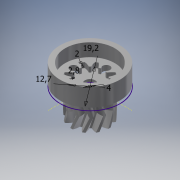
# Autodesk Inventor part: Stirnzahnrad1
Saved by Autodesk Inventor 2019.1 (Build 231200000, 200)
## iProperties
Created: 2018-07-09
Part Number: Stirnzahnrad1
Material: Steel
Document SubType Name: Modeling
Designer: JochenAlt
Categories: <?xml version="1.0" encoding="UTF-16"?> <MemberInstance><Categories><FamilyTemplate><FamilyTemplateParameter ValueType="xs:double" Id="1" ObjectReferenceKey="da_z" ObjectType="kUserParameterObject"/><FamilyTemplateParameter ValueType="xs:double" Id="2" ObjectReferenceKey="da_b" ObjectType="kUserParameterObject"/><FamilyTemplateParameter ValueType="xs:double" Id="3" ObjectReferenceKey="da_beta" ObjectType="kUserParameterObject"/><FamilyTemplateParameter ValueType="xs:double" Id="4" ObjectReferenceKey="da_da" ObjectType="kUserParameterObject"/><FamilyTemplateParameter ValueType="xs:double" Id="5" ObjectReferenceKey="da_aw" ObjectType="kUserParameterObject"/><FamilyTemplateParameter ValueType="xs:string" Id="6" ObjectReferenceKey="EAIAABAAAACIAQAAAAAAAIAAAAAAAAAA" ObjectType="83910656" SubObjectId="SurfaceGeometry"/></FamilyTemplate><ParamToTemplateMap><ParamToTemplate CategoryParameter="//CategoryParameter[@InternalName='046C89C9-8512-4d59-83FE-43B91F4F132A']" TemplateParameter="1"/><ParamToTemplate CategoryParameter="//CategoryParameter[@InternalName='2552DF32-E462-4b46-AEBF-C6C7768E72AC']" TemplateParameter="2"/><ParamToTemplate CategoryParameter="//CategoryParameter[@InternalName='C9EE641D-15FC-4fae-A226-E94C4372FDD7']" TemplateParameter="3"/><ParamToTemplate><ParamToTemplate CategoryParameter="//CategoryParameter[@InternalName='00B6519A-459B-49c7-AD84-2E56D39A5744']" ConstantValue="0.000000"/></ParamToTemplate><ParamToTemplate><ParamToTemplate CategoryParameter="//CategoryParameter[@InternalName='04B31F0E-C7A6-4894-AA32-9629BEFACF47']" ConstantValue="1.000000"/></ParamToTemplate><ParamToTemplate><ParamToTemplate CategoryParameter="//CategoryParameter[@InternalName='43CBEC2E-7847-49e7-A936-2F7889FCB2D9']" ConstantValue="0.250000"/></ParamToTemplate><ParamToTemplate><ParamToTemplate CategoryParameter="//CategoryParameter[@InternalName='B1EFC894-105D-4ebd-86BF-FA20ED196853']" ConstantValue="0.350000"/></ParamToTemplate><ParamToTemplate><ParamToTemplate CategoryParameter="//CategoryParameter[@InternalName='51175063-3D10-4879-93E8-6246FE8B403D']" ConstantValue="2060000000.000000"/></ParamToTemplate><ParamToTemplate><ParamToTemplate CategoryParameter="//CategoryParameter[@InternalName='A3A52E27-4454-46a9-B0BD-C932399B70AF']" ConstantValue="0.300000"/></ParamToTemplate><ParamToTemplate><ParamToTemplate CategoryParameter="//CategoryParameter[@InternalName='91B76062-C214-41d9-B1B9-14D2AB99603D']" ConstantValue="0.100000"/></ParamToTemplate><ParamToTemplate><ParamToTemplate CategoryParameter="//CategoryParameter[@InternalName='374E806E-8B8A-4dda-A9AA-1039D6500AD2']" ConstantValue="10.000000"/></ParamToTemplate><ParamToTemplate><ParamToTemplate CategoryParameter="//CategoryParameter[@InternalName='2D373A89-B862-43d6-8D0B-0CBF12AB9F6C']" ConstantValue="0.349066"/></ParamToTemplate><ParamToTemplate CategoryParameter="//CategoryParameter[@InternalName='37777632-D6A2-4fac-9D53-DB8ACD95C989']" TemplateParameter="4"/><ParamToTemplate CategoryParameter="//CategoryParameter[@InternalName='FD1017F1-B727-4f7e-9707-0F86F1FF9423']" TemplateParameter="5"/><ParamToTemplate><ParamToTemplate CategoryParameter="//CategoryParameter[@InternalName='9E1B4470-B2D3-4ff1-B813-535BB4CDF51A']" ConstantValue="3520000.000000"/></ParamToTemplate><ParamToTemplate><ParamToTemplate CategoryParameter="//CategoryParameter[@InternalName='F8452263-BFF6-458c-9FB1-07C4B99E95CD']" ConstantValue="11400000.000000"/></ParamToTemplate><ParamToTemplate><ParamToTemplate CategoryParameter="//CategoryParameter[@InternalName='3E3BB259-FD49-497f-8171-6EBC954A3479']" ConstantValue="2.000000"/></ParamToTemplate><ParamToTemplate CategoryParameter="//CategoryParameter[@InternalName='27C3BAF2-7550-4e4b-AE2C-0DB134B7D9B7']" TemplateParameter="6"/></ParamToTemplateMap><Category DisplayName="Gear" InternalName="DC85795E-93AB-48d5-8EEE-5A27447B64BD" Mnemonic="Gear"><CategoryParameter DisplayName="z" InternalName="046C89C9-8512-4d59-83FE-43B91F4F132A" Mnemonic="z"/><CategoryParameter DisplayName="b" InternalName="2552DF32-E462-4b46-AEBF-C6C7768E72AC" Mnemonic="b"/><CategoryParameter DisplayName="||b|" InternalName="C9EE641D-15FC-4fae-A226-E94C4372FDD7" Mnemonic="beta"/><CategoryParameter DisplayName="x" InternalName="00B6519A-459B-49c7-AD84-2E56D39A5744" Mnemonic="x"/><CategoryParameter DisplayName="a*" InternalName="04B31F0E-C7A6-4894-AA32-9629BEFACF47" Mnemonic="a"/><CategoryParameter DisplayName="c*" InternalName="43CBEC2E-7847-49e7-A936-2F7889FCB2D9" Mnemonic="c"/><CategoryParameter DisplayName="r|.f|*" InternalName="B1EFC894-105D-4ebd-86BF-FA20ED196853" Mnemonic="rf"/><CategoryParameter DisplayName="E" InternalName="51175063-3D10-4879-93E8-6246FE8B403D" Mnemonic="E"/><CategoryParameter DisplayName="||m|" InternalName="A3A52E27-4454-46a9-B0BD-C932399B70AF" Mnemonic="mi"/><Category DisplayName="SpurGear" InternalName="26C5A22E-A91E-4dfd-A3B3-23CCAFAE1764" Mnemonic="SpurGear"><CategoryParameter DisplayName="m" InternalName="91B76062-C214-41d9-B1B9-14D2AB99603D" Mnemonic="m"/><CategoryParameter DisplayName="P" InternalName="374E806E-8B8A-4dda-A9AA-1039D6500AD2" Mnemonic="PP"/><CategoryParameter DisplayName="||a|" InternalName="2D373A89-B862-43d6-8D0B-0CBF12AB9F6C" Mnemonic="alpha"/><CategoryParameter DisplayName="d|.a|" InternalName="37777632-D6A2-4fac-9D53-DB8ACD95C989" Mnemonic="da"/><CategoryParameter DisplayName="a|.w|" InternalName="FD1017F1-B727-4f7e-9707-0F86F1FF9423" Mnemonic="aw"/><CategoryParameter DisplayName="||s||.Flim|" InternalName="9E1B4470-B2D3-4ff1-B813-535BB4CDF51A" Mnemonic="sFlim"/><CategoryParameter DisplayName="||s||.Hlim|" InternalName="F8452263-BFF6-458c-9FB1-07C4B99E95CD" Mnemonic="sHlim"/><CategoryParameter DisplayName="Typ" InternalName="3E3BB259-FD49-497f-8171-6EBC954A3479" Mnemonic="type"/><CategoryParameter DisplayName="PitchDiameter" InternalName="27C3BAF2-7550-4e4b-AE2C-0DB134B7D9B7" Mnemonic="IDS_PITCHDIAM"/></Category></Category></Categories></MemberInstance>
Density: 1 g/cm^3
Appearance: Steel
CustomPartVersion: 1
Author: JochenAlt
Autodesk Inventor part; units mm, degrees
sketch "Sketch1" plane through (0, 0, 0) normal (0, 0, 1) x (1, 0, 0)
  circle A0 centre (0, 0) radius 7.3851
  dimension "d0" = 14.7701
  constraints: 1 centre point
  measures "d0" diameter of A0
extrude "Extrusion1" add sketch "Sketch1" along normal blind 5.5
ref_plane "Work Plane2" through (0, 0, 2.75) normal (0, 0, 1) x (1, 0, 0)
sketch "Sketch2" plane through (0, 0, 0) normal (0, 0, -1) x (-1, 0, 0)
  circle A0 centre (0, 0) radius 7.3851 projected
  circle A1 centre (0, 0) radius 6.375
  dimension "d3" = 12.75
  constraints: 1 centre point, 1 coincident
  measures "d3" diameter of A1
surface extrude "Flankendurchmesser" sketch "Sketch2" against normal through all shown no curves A1
ref_plane "Work Plane8" through (0, 0, 0) normal (0.9659258, 0.258819, 0) x (0, 0, 1)
ref_plane "Work Plane9" through (0, 0, 0) normal (1, 0, 0) x (0, 1, 0)
spur gear teeth "Stirnzahnrad" teeth 12 pitch diameter 12.7701 tip diameter 14.7701 root diameter 10.2701 face width 5.5 helix angle 20 hand right start plane through (0, 0, 0) normal (0, 0, -1) x (-1, 0, 0)
mirror "Spiegeln2" about plane through (0, 0, 5.5) normal (0, 0, 1)
sketch "Skizze3" plane through (0, 0, 11) normal (0, 0, 1) x (1, 0, 0)
  circle A0 centre (0, 0) radius 2
  circle A1 centre (0, 0) radius 9.6
  circle A2 centre (0, 0) radius 11.6
  circle A3 centre (0, 0) radius 6.35 construction
  circle A4 centre (-6.35, 0) radius 1.4
  circle A5 centre (6.35, 0) radius 1.4
  circle A6 centre (0, 6.35) radius 1.4
  circle A7 centre (0, -6.35) radius 1.4
  line L0 (0, 16.24) -> (0, -16.24) construction
  line L1 (-16.24, 0) -> (16.24, 0) construction
  spline S0 degree 5 poles (-3.3858, 3.8607) (-3.6167, 4.2827) (-3.8063, 4.7273) (-3.9516, 5.1892) (-4.0507, 5.6623) (-4.1029, 6.1405) knots 0 0 0 0 0 0 1 1 1 1 1 1 projected
  spline S1 degree 5 poles (-3.8607, 3.3858) (-3.7721, 3.4869) (-3.6802, 3.585) (-3.585, 3.6802) (-3.4869, 3.7721) (-3.3858, 3.8607) knots 0 0 0 0 0 0 1 1 1 1 1 1 projected
  spline S2 degree 5 poles (-6.1405, 4.1029) (-5.6623, 4.0507) (-5.1892, 3.9516) (-4.7273, 3.8063) (-4.2827, 3.6167) (-3.8607, 3.3858) knots 0 0 0 0 0 0 1 1 1 1 1 1 projected
  arc A8 (-6.1405, 4.1029) -> (-6.6235, 3.2663) centre (0, 0) ccw projected
  spline S3 degree 5 poles (-4.8625, 1.6506) (-5.2735, 1.9006) (-5.66, 2.1909) (-6.0168, 2.5182) (-6.3391, 2.8783) (-6.6235, 3.2663) knots 0 0 0 0 0 0 1 1 1 1 1 1 projected
  spline S4 degree 5 poles (-5.0364, 1.0018) (-5.0102, 1.1337) (-4.9796, 1.2646) (-4.9448, 1.3946) (-4.9058, 1.5233) (-4.8625, 1.6506) knots 0 0 0 0 0 0 1 1 1 1 1 1 projected
  spline S5 degree 5 poles (-7.3693, 0.483) (-6.929, 0.6769) (-6.4698, 0.8276) (-5.9972, 0.9327) (-5.5173, 0.9908) (-5.0364, 1.0018) knots 0 0 0 0 0 0 1 1 1 1 1 1 projected
  arc A9 (-7.3693, 0.483) -> (-7.3693, -0.483) centre (0, 0) ccw projected
  spline S6 degree 5 poles (-5.0364, -1.0018) (-5.5173, -0.9908) (-5.9972, -0.9327) (-6.4698, -0.8276) (-6.929, -0.6769) (-7.3693, -0.483) knots 0 0 0 0 0 0 1 1 1 1 1 1 projected
  spline S7 degree 5 poles (-4.8625, -1.6506) (-4.9058, -1.5233) (-4.9448, -1.3946) (-4.9796, -1.2646) (-5.0102, -1.1337) (-5.0364, -1.0018) knots 0 0 0 0 0 0 1 1 1 1 1 1 projected
  spline S8 degree 5 poles (-6.6235, -3.2663) (-6.3391, -2.8783) (-6.0168, -2.5182) (-5.66, -2.1909) (-5.2735, -1.9006) (-4.8625, -1.6506) knots 0 0 0 0 0 0 1 1 1 1 1 1 projected
  arc A10 (-6.6235, -3.2663) -> (-6.1405, -4.1029) centre (0, 0) ccw projected
  spline S9 degree 5 poles (-3.8607, -3.3858) (-4.2827, -3.6167) (-4.7273, -3.8063) (-5.1892, -3.9516) (-5.6623, -4.0507) (-6.1405, -4.1029) knots 0 0 0 0 0 0 1 1 1 1 1 1 projected
  spline S10 degree 5 poles (-3.3858, -3.8607) (-3.4869, -3.7721) (-3.585, -3.6802) (-3.6802, -3.585) (-3.7721, -3.4869) (-3.8607, -3.3858) knots 0 0 0 0 0 0 1 1 1 1 1 1 projected
  spline S11 degree 5 poles (-4.1029, -6.1405) (-4.0507, -5.6623) (-3.9516, -5.1892) (-3.8063, -4.7273) (-3.6167, -4.2827) (-3.3858, -3.8607) knots 0 0 0 0 0 0 1 1 1 1 1 1 projected
  arc A11 (-4.1029, -6.1405) -> (-3.2663, -6.6235) centre (0, 0) ccw projected
  spline S12 degree 5 poles (-1.6506, -4.8625) (-1.9006, -5.2735) (-2.1909, -5.66) (-2.5182, -6.0168) (-2.8783, -6.3391) (-3.2663, -6.6235) knots 0 0 0 0 0 0 1 1 1 1 1 1 projected
  spline S13 degree 5 poles (-1.0018, -5.0364) (-1.1337, -5.0102) (-1.2646, -4.9796) (-1.3946, -4.9448) (-1.5233, -4.9058) (-1.6506, -4.8625) knots 0 0 0 0 0 0 1 1 1 1 1 1 projected
  spline S14 degree 5 poles (-0.483, -7.3693) (-0.6769, -6.929) (-0.8276, -6.4698) (-0.9327, -5.9972) (-0.9908, -5.5173) (-1.0018, -5.0364) knots 0 0 0 0 0 0 1 1 1 1 1 1 projected
  arc A12 (-0.483, -7.3693) -> (0.483, -7.3693) centre (0, 0) ccw projected
  spline S15 degree 5 poles (1.0018, -5.0364) (0.9908, -5.5173) (0.9327, -5.9972) (0.8276, -6.4698) (0.6769, -6.929) (0.483, -7.3693) knots 0 0 0 0 0 0 1 1 1 1 1 1 projected
  spline S16 degree 5 poles (1.6506, -4.8625) (1.5233, -4.9058) (1.3946, -4.9448) (1.2646, -4.9796) (1.1337, -5.0102) (1.0018, -5.0364) knots 0 0 0 0 0 0 1 1 1 1 1 1 projected
  spline S17 degree 5 poles (3.2663, -6.6235) (2.8783, -6.3391) (2.5182, -6.0168) (2.1909, -5.66) (1.9006, -5.2735) (1.6506, -4.8625) knots 0 0 0 0 0 0 1 1 1 1 1 1 projected
  arc A13 (3.2663, -6.6235) -> (4.1029, -6.1405) centre (0, 0) ccw projected
  spline S18 degree 5 poles (3.3858, -3.8607) (3.6167, -4.2827) (3.8063, -4.7273) (3.9516, -5.1892) (4.0507, -5.6623) (4.1029, -6.1405) knots 0 0 0 0 0 0 1 1 1 1 1 1 projected
  spline S19 degree 5 poles (3.8607, -3.3858) (3.7721, -3.4869) (3.6802, -3.585) (3.585, -3.6802) (3.4869, -3.7721) (3.3858, -3.8607) knots 0 0 0 0 0 0 1 1 1 1 1 1 projected
  spline S20 degree 5 poles (6.1405, -4.1029) (5.6623, -4.0507) (5.1892, -3.9516) (4.7273, -3.8063) (4.2827, -3.6167) (3.8607, -3.3858) knots 0 0 0 0 0 0 1 1 1 1 1 1 projected
  arc A14 (6.1405, -4.1029) -> (6.6235, -3.2663) centre (0, 0) ccw projected
  spline S21 degree 5 poles (4.8625, -1.6506) (5.2735, -1.9006) (5.66, -2.1909) (6.0168, -2.5182) (6.3391, -2.8783) (6.6235, -3.2663) knots 0 0 0 0 0 0 1 1 1 1 1 1 projected
  spline S22 degree 5 poles (5.0364, -1.0018) (5.0102, -1.1337) (4.9796, -1.2646) (4.9448, -1.3946) (4.9058, -1.5233) (4.8625, -1.6506) knots 0 0 0 0 0 0 1 1 1 1 1 1 projected
  spline S23 degree 5 poles (7.3693, -0.483) (6.929, -0.6769) (6.4698, -0.8276) (5.9972, -0.9327) (5.5173, -0.9908) (5.0364, -1.0018) knots 0 0 0 0 0 0 1 1 1 1 1 1 projected
  arc A15 (7.3693, -0.483) -> (7.3693, 0.483) centre (0, 0) ccw projected
  spline S24 degree 5 poles (5.0364, 1.0018) (5.5173, 0.9908) (5.9972, 0.9327) (6.4698, 0.8276) (6.929, 0.6769) (7.3693, 0.483) knots 0 0 0 0 0 0 1 1 1 1 1 1 projected
  spline S25 degree 5 poles (4.8625, 1.6506) (4.9058, 1.5233) (4.9448, 1.3946) (4.9796, 1.2646) (5.0102, 1.1337) (5.0364, 1.0018) knots 0 0 0 0 0 0 1 1 1 1 1 1 projected
  spline S26 degree 5 poles (6.6235, 3.2663) (6.3391, 2.8783) (6.0168, 2.5182) (5.66, 2.1909) (5.2735, 1.9006) (4.8625, 1.6506) knots 0 0 0 0 0 0 1 1 1 1 1 1 projected
  arc A16 (6.6235, 3.2663) -> (6.1405, 4.1029) centre (0, 0) ccw projected
  spline S27 degree 5 poles (3.8607, 3.3858) (4.2827, 3.6167) (4.7273, 3.8063) (5.1892, 3.9516) (5.6623, 4.0507) (6.1405, 4.1029) knots 0 0 0 0 0 0 1 1 1 1 1 1 projected
  spline S28 degree 5 poles (3.3858, 3.8607) (3.4869, 3.7721) (3.585, 3.6802) (3.6802, 3.585) (3.7721, 3.4869) (3.8607, 3.3858) knots 0 0 0 0 0 0 1 1 1 1 1 1 projected
  spline S29 degree 5 poles (4.1029, 6.1405) (4.0507, 5.6623) (3.9516, 5.1892) (3.8063, 4.7273) (3.6167, 4.2827) (3.3858, 3.8607) knots 0 0 0 0 0 0 1 1 1 1 1 1 projected
  arc A17 (4.1029, 6.1405) -> (3.2663, 6.6235) centre (0, 0) ccw projected
  spline S30 degree 5 poles (1.6506, 4.8625) (1.9006, 5.2735) (2.1909, 5.66) (2.5182, 6.0168) (2.8783, 6.3391) (3.2663, 6.6235) knots 0 0 0 0 0 0 1 1 1 1 1 1 projected
  spline S31 degree 5 poles (1.0018, 5.0364) (1.1337, 5.0102) (1.2646, 4.9796) (1.3946, 4.9448) (1.5233, 4.9058) (1.6506, 4.8625) knots 0 0 0 0 0 0 1 1 1 1 1 1 projected
  spline S32 degree 5 poles (0.483, 7.3693) (0.6769, 6.929) (0.8276, 6.4698) (0.9327, 5.9972) (0.9908, 5.5173) (1.0018, 5.0364) knots 0 0 0 0 0 0 1 1 1 1 1 1 projected
  arc A18 (0.483, 7.3693) -> (-0.483, 7.3693) centre (0, 0) ccw projected
  spline S33 degree 5 poles (-1.0018, 5.0364) (-0.9908, 5.5173) (-0.9327, 5.9972) (-0.8276, 6.4698) (-0.6769, 6.929) (-0.483, 7.3693) knots 0 0 0 0 0 0 1 1 1 1 1 1 projected
  spline S34 degree 5 poles (-1.6506, 4.8625) (-1.5233, 4.9058) (-1.3946, 4.9448) (-1.2646, 4.9796) (-1.1337, 5.0102) (-1.0018, 5.0364) knots 0 0 0 0 0 0 1 1 1 1 1 1 projected
  spline S35 degree 5 poles (-3.2663, 6.6235) (-2.8783, 6.3391) (-2.5182, 6.0168) (-2.1909, 5.66) (-1.9006, 5.2735) (-1.6506, 4.8625) knots 0 0 0 0 0 0 1 1 1 1 1 1 projected
  arc A19 (-3.2663, 6.6235) -> (-4.1029, 6.1405) centre (0, 0) ccw projected
  point P0 (0, 0)
  dimension "d49" = 19.2
  dimension "d50" = 2
  dimension "d51" = 12.7
  dimension "d52" = 2.8
  dimension "d53" = 4
  constraints: 8 centre point, 4 coincident, 4 point on circle, 4 point on line, 3 equal radius, 36 other
  measures "d49" diameter of A1
  measures "d50" radial gap between concentric circles of A2 A1
  measures "d51" diameter of A3
  measures "d52" diameter of A4
  measures "d53" diameter of A0
extrude "Extrusion6" add sketch "Skizze3" along normal blind 1 contours A4 S6 A9 S5 | A4 S5 S4 S3 A8 S2 S1 S0 A19 S35 S34 S33 A6 S32 S31 S30 A17 S29 S28 S27 A16 S26 S25 S24 A5 S23 S22 S21 A14 S20 S19 S18 A13 S17 S16 S15 A7 S14 S13 S12 A11 S11 S10 S9 A10 S8 S7 S6 | S33 A18 S32 A6 | A7 S15 A12 S14 | S24 A15 S23 A5 picked at (-5.7175, 0.0227) picked at (-0.0292, 5.7204) picked at (0.0292, -5.7204) picked at (5.7204, 0.0292)
extrude "Extrusion2" add sketch "Skizze3" along normal blind 2 from surface at 1 contours A1 | A2
extrude "Extrusion3" add sketch "Skizze3" along normal blind 5 from surface at 3 contours A2
extrude "Extrusion4" cut sketch "Skizze3" against normal through all contours A0
sketch "Skizze5" plane through (0, 0, 0) normal (0, 0, -1) x (-1, 0, 0)
  circle A0 centre (0, 0) radius 9.6 projected
extrude "Extrusion5" add sketch "Skizze5" against normal blind 0.5 separate body
combine bodies "Kombinieren1" operation type subtract main body 1 bodies to subtract 2
sketch "Skizze6" plane through (0.6223, 6.2358, 0.5) normal (0, 0, -1) x (-0.9033557, -0.4288921, 0)
  circle A0 centre (3.2366, -5.3663) radius 5.1351 construction
  dimension "d62" = 10.2701
  constraints: 1 coincident, 4 other
equation "\"d0\" = da_da"
equation "\"d1\" = da_b"
equation "\"d3\" = da_dw"
equation "\"d16\" = da_aw"
equation "\"d43\" = da_aw"
equation "\"d46\" = da_aw"
equation "\"da_da\" = 14.770133"
equation "\"da_b\" = 5.5"
equation "\"da_dw\" = 12.75"
equation "\"da_aw\" = 25.5"
body "Solid1"
body "Srf1"
